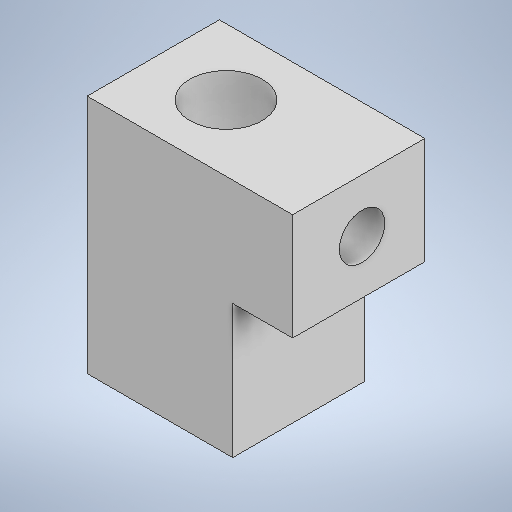
# Autodesk Inventor part: motor_rubik_adapter
Saved by Autodesk Inventor 2025 (Build 290162010, 162A)
## iProperties
Created: 2025-02-10
Part Number: motor_rubik_adapter
Material: Generic
Document SubType Name: Modeling
Designer: aduwa
Density: 1 g/cm^3
Appearance: Default
Author: aduwa
Autodesk Inventor part; units mm, degrees
ref_plane "YZ Plane" through (0, 0, 0) normal (1, 0, 0) x (0, 1, 0)
ref_plane "XZ Plane" through (0, 0, 0) normal (0, 1, 0) x (-1, 0, 0)
ref_plane "XY Plane" through (0, 0, 0) normal (0, 0, 1) x (1, 0, 0)
sketch "Sketch1" plane through (0, 0, 0) normal (0, 1, 0) x (-1, 0, 0)
  circle A0 centre (0, 0) radius 2.7
  line L0 (5.45, 4.95) -> (-5.45, 4.95)
  line L1 (-5.45, 4.95) -> (-5.45, -4.95)
  line L2 (-5.45, -4.95) -> (5.45, -4.95)
  line L3 (5.45, -4.95) -> (5.45, 4.95)
  line L4 (5.45, 4.95) -> (-5.45, -4.95) construction
  line L5 (-5.45, 4.95) -> (5.45, -4.95) construction
  dimension "d0" = 5.4
  dimension "d1" = 10.9
  dimension "d2" = 9.9
  constraints: 12 end point, 2 midpoint, 2 parallel, 1 centre point, 1 coincident, 1 horizontal, 1 perpendicular
  measures "d0" diameter of A0
  measures "d1" distance of L2.end L1.end
  measures "d2" distance of L1.end L0.end
extrude "Extrusion1" add sketch "Sketch1" along normal blind 18
sketch "Sketch2" plane through (5.45, 0, 4.95) normal (1, 0, 0) x (0, 0, -1)
  circle A0 centre (5.2, 14) radius 1.7
  line L0 (0, 18) -> (9.9, 18) projected
  point P0 (4.95, 0)
  dimension "d5" = 4
  dimension "d6" = 3.4
  constraints: 1 centre point
  measures "d5" distance from line of L0 A0.centre
  measures "d6" diameter of A0
extrude "Extrusion2" cut sketch "Sketch2" against normal blind 5
sketch "Sketch3" plane through (5.45, 0, 4.95) normal (1, 0, 0) x (0, 0, -1)
  line L0 (0, 0) -> (0, 18) projected
  line L1 (9.9, 0) -> (9.9, 18) projected
  line L2 (0, 18) -> (9.9, 18)
  line L3 (9.9, 18) -> (9.9, 10)
  line L4 (9.9, 10) -> (0, 10)
  line L5 (0, 10) -> (0, 18)
  circle A0 centre (5.2, 14) radius 1.7 projected
  point P0 (4.95, 0)
  dimension "d9" = 8
  constraints: 8 end point, 2 parallel, 1 horizontal, 1 perpendicular, 1 point on line
  measures "d9" distance of L2.end L3.end
extrude "Extrusion3" add sketch "Sketch3" along normal blind 4.489
body "Solid1"
